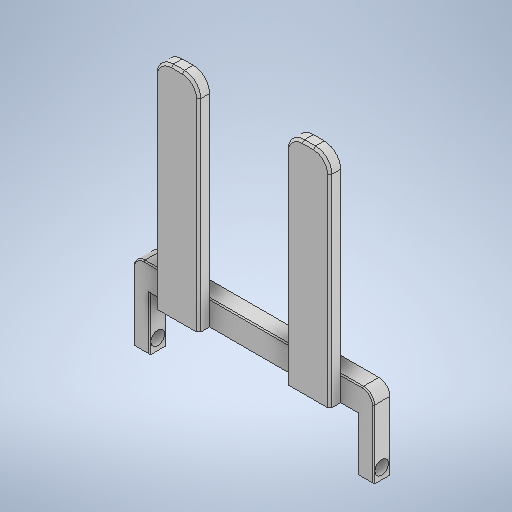
# Autodesk Inventor part: Fork
Saved by Autodesk Inventor 2025.2 (Build 292293000, 293)
## iProperties
Created: 2025-01-08
Part Number: Fork
Material: Generic
Document SubType Name: Modeling
Designer: Sergio Quintero
Density: 1 g/cm^3
Appearance: Default
Author: Sergio Quintero
Autodesk Inventor part; units mm, degrees
ref_plane "YZ Plane" through (0, 0, 0) normal (1, 0, 0) x (0, 1, 0)
ref_plane "XZ Plane" through (0, 0, 0) normal (0, 1, 0) x (-1, 0, 0)
ref_plane "XY Plane" through (0, 0, 0) normal (0, 0, 1) x (1, 0, 0)
sketch "Sketch1" plane through (0, 0, 0) normal (0, 0, 1) x (1, 0, 0)
  line L0 (-220, 72.5) -> (220, 72.5)
  line L1 (220, 72.5) -> (220, -72.5)
  line L2 (220, -72.5) -> (-220, -72.5)
  line L3 (-220, -72.5) -> (-220, 72.5)
  line L4 (-220, 72.5) -> (220, -72.5) construction
  line L5 (220, 72.5) -> (-220, -72.5) construction
  point P0 (0, 0)
  dimension "d0" = 440
  dimension "d1" = 145
  constraints: 12 end point, 2 midpoint, 2 parallel, 1 horizontal, 1 perpendicular
  measures "d0" distance of L1.end L2.end
  measures "d1" distance of L0.end L1.end
extrude "Extrusion1" add sketch "Sketch1" along normal blind 30
sketch "Sketch2" plane through (0, 0, 30) normal (0, 0, 1) x (1, 0, 0)
  line L0 (-220, -72.5) -> (220, -72.5) projected
  line L1 (-190, -72.5) -> (190, -72.5)
  line L2 (190, -72.5) -> (190, 27.5)
  line L3 (190, 27.5) -> (-190, 27.5)
  line L4 (-190, 27.5) -> (-190, -72.5)
  line L5 (220, -72.5) -> (220, 72.5) projected
  line L6 (0, 72.5) -> (0, -72.5) construction
  line L7 (220, 72.5) -> (-220, 72.5) construction
  point P0 (0, 0)
  dimension "d4" = 30
  dimension "d5" = 45
  constraints: 10 end point, 2 parallel, 2 perpendicular, 1 horizontal, 1 midpoint, 1 point on line, 1 other
  measures "d4" distance between parallel lines of L5 L2
  measures "d5" distance between parallel lines of L7 L3
extrude "Extrusion2" cut sketch "Sketch2" against normal blind 30
fillet "Fillet1" radius 20 2 edges at (220, 72.5, 15) (-220, 72.5, 15)
sketch "Sketch3" plane through (0, 0, 30) normal (0, 0, 1) x (1, 0, 0)
  line L0 (-190, 27.5) -> (190, 27.5) projected
  line L1 (-160, 27.5) -> (-80, 27.5)
  line L2 (-80, 27.5) -> (-80, 427.5)
  line L3 (-80, 427.5) -> (-160, 427.5)
  line L4 (-160, 427.5) -> (-160, 27.5)
  line L5 (-220, 52.5) -> (-220, -72.5) projected
  line L6 (-220, -72.5) -> (-190, -72.5) projected
  point P0 (0, 0)
  point P1 (-205, -72.5)
  dimension "d9" = 60
  dimension "d10" = 80
  dimension "d11" = 500
  constraints: 8 end point, 2 parallel, 1 horizontal, 1 midpoint, 1 perpendicular, 1 point on line
  measures "d9" distance between parallel lines of L4 L5
  measures "d10" distance between parallel lines of L2 L4
  measures "d11" distance from line of point (-205, -72.5) L3
extrude "Extrusion3" add sketch "Sketch3" along normal blind 20 separate body
fillet "Fillet2" radius 30 2 edges at (-160, 427.5, 40) (-80, 427.5, 40)
chamfer "Chamfer1" distance 4 angle 45 5 edges at (-151.2132, 418.7132, 50) (-120, 427.5, 50) (-88.7868, 418.7132, 50) (-80, 212.5, 50) (-160, 212.5, 50)
mirror "Mirror1" about plane through (0, 0, 0) normal (1, 0, 0) of "Extrusion3", "Fillet2", "Chamfer1" bodies 2
chamfer "Chamfer2" distance 2 angle 45 9 edges at (-190, -22.5, 30) (-205, -72.5, 30) (-220, -10, 30) (-214.1421, 66.6421, 30) (0, 72.5, 30) (214.1421, 66.6421, 30) (220, -10, 30) (190, -22.5, 30) (205, -72.5, 30)
sketch "Sketch4" plane through (-190, -72.5, 0) normal (1, 0, 0) x (0, 0, -1)
  line L0 (0, 0) -> (-28, 0) construction
  line L1 (0, 100) -> (0, 0) construction
  point P0 (0, 72.5)
  point P1 (-15, 20)
  point P2 (-14, 0)
  dimension "d21" = 20
  dimension "d22" = 15
  constraints: 1 midpoint
  measures "d21" vertical distance of point (-14, 0) point (-15, 20)
  measures "d22" distance from line of L1 point (-15, 20)
hole "Hole1" at (-190, -52.5, 15) direction (-1, 0, 0) diameter 25 end through all bodies 1
mirror "Mirror2" about plane through (0, 0, 0) normal (1, 0, 0) of "Hole1" bodies 1
body "Solid1"
body "Solid2"
